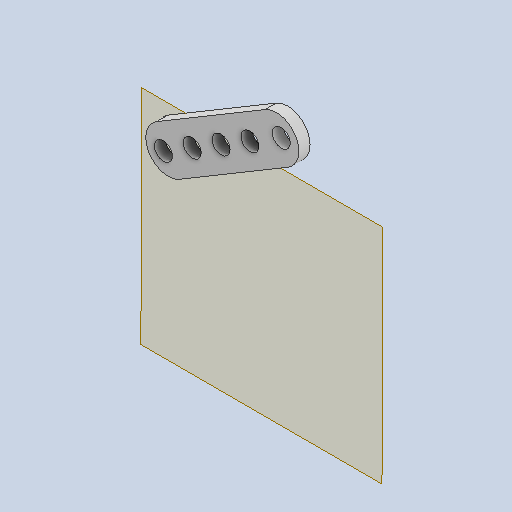
# Autodesk Inventor part: vertex-arm
Saved by Autodesk Inventor 2024.1 (Build 281209000, 209)
## iProperties
Created: 2025-06-12
Part Number: vertex-arm
Material: Generic
Document SubType Name: Modeling
Designer: iwheard
Density: 1 g/cm^3
Appearance: Default
Author: iwheard
Autodesk Inventor part; units mm, degrees
ref_plane "YZ Plane" through (0, 0, 0) normal (1, 0, 0) x (0, 1, 0)
ref_plane "XZ Plane" through (0, 0, 0) normal (0, 1, 0) x (-1, 0, 0)
ref_plane "XY Plane" through (0, 0, 0) normal (0, 0, 1) x (1, 0, 0)
ref_plane "Work Plane1" through (-0.0283, 0.0058, 0) normal (0, 0, 1) x (1, -0.0011, 0)
sketch "Sketch1" plane through (-0.0283, 0.0058, 0) normal (0, 0, 1) x (1, -0.0011, 0)
  circle A0 centre (-15.5573, 14.0686) radius 1.6 projected
  line L0 (-16.0804, 9.0961) -> (-20.1845, 15.9631)
  line L1 (-20.1845, 15.9631) -> (6.0115, 31.6191)
  line L2 (6.0115, 31.6191) -> (10.1156, 24.7521)
  line L3 (10.1156, 24.7521) -> (-16.0804, 9.0961)
  circle A1 centre (5.4884, 26.6466) radius 1.6 projected
  circle A2 centre (-15.5573, 14.0686) radius 1.6
  circle A3 centre (5.4884, 26.6466) radius 1.6
  circle A4 centre (-10.407, 17.1467) radius 1.6
  circle A5 centre (-5.2567, 20.2248) radius 1.6
  circle A6 centre (-0.1064, 23.3028) radius 1.6
  point P0 (0.0283, -0.0058)
  dimension "d0" = 4
  dimension "d1" = 8
  dimension "d2" = 3
  dimension "d3" = 3
  dimension "d4" = 4
  dimension "d7" = 6
  constraints: 8 end point, 5 centre point, 2 coincident, 2 concentric, 2 parallel, 1 perpendicular, 7 other
  measures "d0" distance from line of L3 A0.centre
  measures "d1" distance between parallel lines of L1 L3
  measures "d2" distance from line of L0 A0.centre
  measures "d3" distance from line of L2 A1.centre
  measures "d4" distance from line of L3 A1.centre
  measures "d7" distance of A2.centre A4.centre
extrude "Extrusion1" add sketch "Sketch1" along normal blind 2
fillet "Fillet1" radius 4 4 edges at (-20.1958, 15.9904, 1) (-16.099, 9.119, 1) (6.0167, 31.6186, 1) (10.1135, 24.7472, 1)
body "Solid1"
